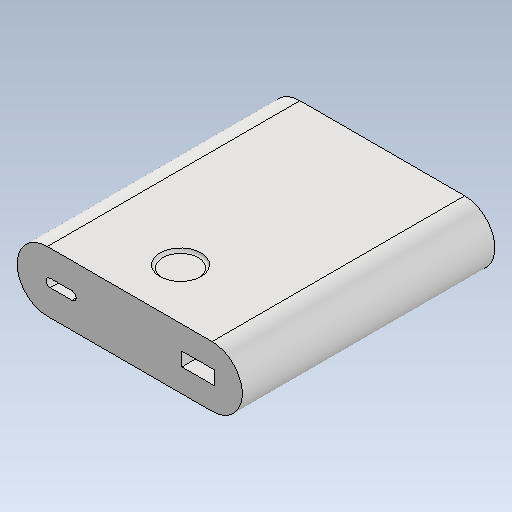
# Autodesk Inventor part: power-bank
Saved by Autodesk Inventor 2025 (Build 290162000, 162)
## iProperties
Created: 2025-08-23
Part Number: power-bank
Material: Generic
Document SubType Name: Modeling
Designer: HP
Density: 1 g/cm^3
Appearance: Default
Author: HP
Autodesk Inventor part; units mm, degrees
ref_plane "YZ Plane" through (0, 0, 0) normal (1, 0, 0) x (0, 1, 0)
ref_plane "XZ Plane" through (0, 0, 0) normal (0, 1, 0) x (-1, 0, 0)
ref_plane "XY Plane" through (0, 0, 0) normal (0, 0, 1) x (1, 0, 0)
sketch "Sketch1" plane through (0, 0, 0) normal (0, 0, 1) x (1, 0, 0)
  line L0 (-30, 0) -> (30, 0) construction
  line L1 (-30, -11) -> (30, -11)
  line L2 (30, 11) -> (-30, 11)
  arc A0 (-30, 11) -> (-30, -11) centre (-30, 0) ccw
  arc A1 (30, -11) -> (30, 11) centre (30, 0) ccw
  point P0 (0, 0)
  point P1 (0, 0)
  dimension "d0" = 22
  dimension "d1" = 60
  constraints: 8 end point, 4 point on circle, 4 tangent, 2 centre point, 1 coincident, 1 horizontal, 1 midpoint, 1 parallel
  measures "d0" diameter of A1
  measures "d1" distance of L0.start L0.end
extrude "Extrusion1" add sketch "Sketch1" along normal mid plane 92
sketch "Sketch2" plane through (0, 0, 46) normal (0, 0, 1) x (1, 0, 0)
  line L0 (19, 2.5) -> (31, 2.5)
  line L1 (31, 2.5) -> (31, -2.5)
  line L2 (31, -2.5) -> (19, -2.5)
  line L3 (19, -2.5) -> (19, 2.5)
  line L4 (19, 2.5) -> (31, -2.5) construction
  line L5 (31, 2.5) -> (19, -2.5) construction
  arc A0 (30, -11) -> (30, 11) centre (30, 0) ccw projected
  line L6 (30, 11) -> (-30, 11) projected
  arc A1 (-30, 11) -> (-30, -11) centre (-30, 0) ccw projected
  line L7 (-30, -11) -> (30, -11) projected
  line L8 (-29, 0) -> (-21, 0) construction
  line L9 (-29, -1.5) -> (-21, -1.5)
  line L10 (-21, 1.5) -> (-29, 1.5)
  arc A2 (-29, 1.5) -> (-29, -1.5) centre (-29, 0) ccw
  arc A3 (-21, -1.5) -> (-21, 1.5) centre (-21, 0) ccw
  point P0 (0, 0)
  point P1 (25, 0)
  point P2 (-25, 0)
  dimension "d4" = 5
  dimension "d5" = 12
  dimension "d6" = 25
  dimension "d13" = 3
  dimension "d14" = 8
  dimension "d15" = 25
  constraints: 20 end point, 4 point on circle, 4 tangent, 3 midpoint, 3 parallel, 2 centre point, 2 horizontal, 2 horizontal alignment, 1 perpendicular
  measures "d4" distance between parallel lines of L2 L0
  measures "d5" distance between parallel lines of L1 L3
  measures "d6" distance of point (25, 0) point (0, 0)
  measures "d13" diameter of A3
  measures "d14" distance of L8.start L8.end
  measures "d15" distance of point (0, 0) point (-25, 0)
extrude "Extrusion2" cut sketch "Sketch2" against normal blind 10 contours L0 L1 L2 L3 | A2 L10 A3 L9
sketch "Sketch3" plane through (-30, 11, 46) normal (0, 1, 0) x (1, 0, 0)
  circle A0 centre (30, 18.5011) radius 7.5
  point P0 (30, 46)
  dimension "d9" = 15
  constraints: 1 centre point
  measures "d9" diameter of A0
extrude "Extrusion3" cut sketch "Sketch3" against normal blind 1
fillet "Fillet1" radius 1 1 edges at (-7.5, 10, 27.4989)
body "Solid1"
